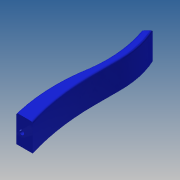
# Autodesk Inventor part: UA-70 Denkmal2
Saved by Autodesk Inventor 2014 (Build 180170000, 170)
## iProperties
Created: 2014-07-02
Part Number: UA-70 Denkmal2
Material: Allgemein
Document SubType Name: Modeling
Designer: Semenov
Density: 1 g/cm^3
Appearance: Vorgabe
Author: Semenov
Autodesk Inventor part; units mm, degrees
ref_plane "YZ Plane" through (0, 0, 0) normal (1, 0, 0) x (0, 1, 0)
ref_plane "XZ Plane" through (0, 0, 0) normal (0, 1, 0) x (-1, 0, 0)
ref_plane "XY Plane" through (0, 0, 0) normal (0, 0, 1) x (1, 0, 0)
sketch "Skizze3" plane through (0, 0, 0) normal (0, 0, 1) x (1, 0, 0)
  line L0 (-225, 400) -> (225, 400)
  line L1 (225, 400) -> (225, -400)
  line L2 (225, -400) -> (-225, -400)
  line L3 (-225, -400) -> (-225, 400)
  arc A0 (-195.1149, 0) -> (-225, -400) centre (2466.8593, -400) ccw
  arc A1 (-195.1149, 0) -> (-195, 270) centre (-1096.0822, 135.3833) ccw
  arc A2 (225, -400) -> (191.0498, 0) centre (-2148.3658, -400) ccw
  arc A3 (195, 400) -> (191.0498, 0) centre (1296.9948, 189.0977) ccw
  arc A4 (195, 400) -> (-98.428, 330) centre (195, -250) ccw
  arc A5 (-112.8051, 0) -> (-95, -400) centre (880.9564, -156.1612) ccw
  arc A6 (-112.8051, 0) -> (-145, 340) centre (-793.9104, 107.0299) ccw
  arc A7 (-135, 310) -> (-195, 270) centre (195, -250) ccw
  arc A8 (-65, 0) -> (-5, -400) centre (1298.3333, 0) ccw
  arc A9 (-98.428, 330) -> (-135, 310) centre (195, -250) ccw construction
  line L4 (-65, 0) -> (-65, 238.5671) construction
  arc A10 (-65, 142.5015) -> (-115, 370) centre (-607.5556, 142.5015) ccw
  line L5 (-65, 142.5015) -> (-65, 0)
  arc A11 (-115, 370) -> (-145, 340) centre (-60.8986, 285.8986) ccw
  arc A12 (-98.428, 330) -> (-225, 400) centre (-144761.9711, -261097.0223) ccw construction
  arc A13 (175.6814, 150) -> (-98.428, 330) centre (-1149.0878, -1568.6875) ccw construction
  point P0 (0, 0)
  point P1 (-225.0722, 0)
  point P2 (0, 400.05)
  point P3 (-225, 0)
  point P4 (0, 400)
  dimension "d5" = 800
  dimension "d8" = 450
  dimension "d9" = 670
  dimension "d10" = 30
  dimension "d11" = 40
  dimension "d12" = 30
  dimension "d14" = 50
  dimension "d16" = 130
  dimension "d18" = 90
  dimension "d19" = 740
  dimension "d21" = 90
  dimension "d22" = 230
  dimension "d23" = 140
  dimension "d26" = 100
  dimension "d28" = 730
  dimension "d34" = 160
  dimension "d35" = 30
  dimension "d36" = 770
  dimension "d38" = 100
  dimension "d51" = 323.428
  dimension "d52" = 250
  dimension "d53" = 2170
  constraints: 32 point on circle, 14 centre point, 12 end point, 12 tangent, 6 horizontal alignment, 4 point on line, 3 parallel, 2 midpoint, 2 vertical alignment, 1 collinear, 1 horizontal, 1 perpendicular
  measures "d5" distance of L2.end L0.start
  measures "d8" distance of L0.start L0.end
  measures "d9" distance from line of A1.end L2
  measures "d10" distance from line of A1.end L3
  measures "d11" distance edge to line of A1 L3
  measures "d12" distance from line of A3.start L1
  measures "d14" distance edge to line of A3 L1
  measures "d16" distance from line of A5.end L3
  measures "d18" distance from line of A7.start L3
  measures "d19" distance from line of A6.end L2
  measures "d21" distance of A8.end A5.end
  measures "d22" distance from line of L1 A8.end
  measures "d23" horizontal distance of A8.end A6.end
  measures "d26" distance edge to line of A5 L3
  measures "d28" distance from line of A4.end L2
  measures "d34" distance between parallel lines of L4 L3
  measures "d35" horizontal distance of A10.end A6.end
  measures "d36" distance from line of L2 A10.end
  measures "d38" radius of A11
  measures "d51" distance from line of A4.end L1
  measures "d52" distance from line of A13.start L0
  measures "d53" radius of A13
extrude "Extrusion3" add sketch "Skizze3" against normal blind 150 contours A10 L5 A8 L2 A5 A6 A11
fillet "Rundung1" radius 10 8 edges at (-65, 71.2508, 0) (-49.9166, -202.2375, 0) (-106.3148, 350.1654, 0) (-73.4224, 237.729, 0) (-124.0049, -200.8948, 0) (-106.2073, 156.2669, 0) (-139.828, 325.0573, 0) (-131.6093, 356.6093, 0)
sketch "Skizze8" plane through (-95, -400, -150) normal (0, -1, 0) x (1, 0, 0)
  line L0 (0, 140) -> (0, 0) projected
  line L1 (90, 0) -> (0, 0) projected
  circle A0 centre (30, 70) radius 12.5
  point P0 (95, 150)
  dimension "d62" = 25
  dimension "d63" = 70
  dimension "d64" = 30
  constraints: 1 centre point
  measures "d62" diameter of A0
  measures "d63" distance from line of A0.centre L1
  measures "d64" distance from line of A0.centre L0
extrude "Extrusion4" cut sketch "Skizze8" against normal blind 100
